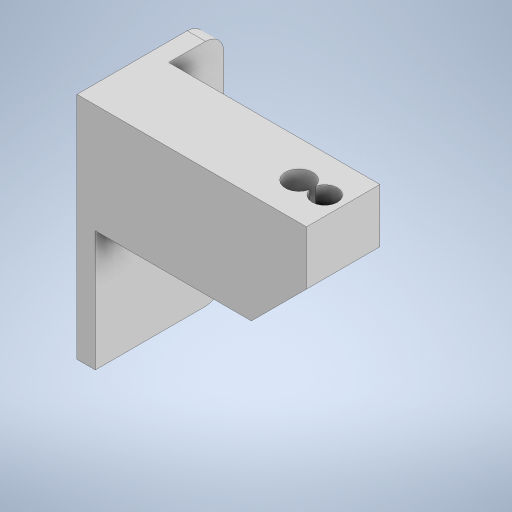
# Autodesk Inventor part: Futaba Antenna Mount
Saved by Autodesk Inventor 2024 (Build 280153000, 153)
## iProperties
Created: 2023-11-29
Part Number: Futaba Antenna Mount
Material: Generic
Document SubType Name: Modeling
Designer: close
Density: 1 g/cm^3
Appearance: Default
Author: close
Autodesk Inventor part; units mm, degrees
ref_plane "YZ Plane" through (0, 0, 0) normal (1, 0, 0) x (0, 1, 0)
ref_plane "XZ Plane" through (0, 0, 0) normal (0, 1, 0) x (-1, 0, 0)
ref_plane "XY Plane" through (0, 0, 0) normal (0, 0, 1) x (1, 0, 0)
sketch "Sketch1" plane through (0, 0, 0) normal (1, 0, 0) x (0, 1, 0)
  line L0 (0, 0) -> (25, 0)
  line L1 (25, 0) -> (25, -8)
  line L2 (25, -8) -> (0, -8)
  line L3 (0, -8) -> (0, 0)
  line L4 (25, -8) -> (12.5, -8)
  line L5 (12.5, -8) -> (12.5, -14)
  line L6 (12.5, -14) -> (25, -14)
  line L7 (25, -14) -> (25, -8)
  line L8 (0, -8) -> (12.5, -8)
  line L9 (12.5, -8) -> (12.5, -14)
  line L10 (12.5, -14) -> (0, -14)
  line L11 (0, -14) -> (0, -8)
  line L12 (25, 0) -> (13.125, 0)
  line L13 (13.125, 0) -> (13.125, -8)
  line L14 (13.125, -8) -> (25, -8)
  line L15 (25, -8) -> (25, 0)
  line L16 (19.5, -11) -> (5.5, -11) construction
  circle A0 centre (19.5, -11) radius 1.65
  circle A1 centre (5.5, -11) radius 1.65
  circle A2 centre (12.5, -11) radius 1.336701
  point P0 (12.5, -8)
  point P1 (25, -11)
  point P2 (12.5, -8)
  point P3 (12.5, -8)
  point P4 (13.125, 0)
  dimension "d0" = 0.625
  dimension "d1" = 14
  dimension "d2" = 25
  dimension "d3" = 12.5
  dimension "d4" = 12.5
  dimension "d6" = 3
  dimension "d7" = 0
  dimension "d8" = 8
  dimension "d11" = 3.3
  dimension "d12" = 3.3
  dimension "d28" = 5.5
  constraints: 34 end point, 8 parallel, 5 horizontal, 4 perpendicular, 3 centre point, 3 midpoint, 2 coincident, 1 collinear, 1 point on line
  measures "d0" distance from line of L13 point (12.5, -8)
  measures "d1" distance of L16.start L16.end
  measures "d2" distance between parallel lines of L3 L1
  measures "d3" distance between parallel lines of L7 L5
  measures "d4" distance between parallel lines of L11 L9
  measures "d6" distance from line of L16.start L6
  measures "d7" distance from line of point (25, -11) L16
  measures "d8" distance between parallel lines of L0 L2
  measures "d11" diameter of A0
  measures "d12" diameter of A1
  measures "d28" distance of point (25, -11) L16.start
sketch "Sketch1 outline for Extrusion1" plane through (0, 0, 0) normal (1, 0, 0) x (0, 1, 0)
  line L0 (0, 0) -> (0, -8)
  line L1 (25, 0) -> (0, 0)
  line L2 (0, -8) -> (0, -14)
  line L3 (25, -8) -> (25, 0)
  line L4 (0, -14) -> (12.5, -14)
  line L5 (25, -14) -> (25, -8)
  line L6 (12.5, -14) -> (25, -14)
  circle A0 centre (5.5, -11) radius 1.65
  circle A1 centre (12.5, -11) radius 1.336701
  circle A2 centre (19.5, -11) radius 1.65
extrude "Extrusion1" add sketch "Sketch1 outline for Extrusion1" along normal blind 2
fillet "Fillet1" radius 2 3 edges at (1, 25, -14) (1, 12.5, -14) (1, 0, -14)
sketch "Sketch1 outline for Extrusion2" plane through (0, 0, 0) normal (1, 0, 0) x (0, 1, 0)
  line L0 (13.125, 0) -> (13.125, -8)
  line L1 (25, 0) -> (13.125, 0)
  line L2 (25, -8) -> (25, 0)
  line L3 (13.125, -8) -> (25, -8)
extrude "Extrusion2" add sketch "Sketch1 outline for Extrusion2" along normal blind 25
chamfer "Chamfer1" distance 6 angle 45 1 edges at (25, 13.125, -4)
sketch "Sketch2" plane through (0, 25, 0) normal (0, 1, 0) x (1, 0, 0)
  line L0 (20.2, 4) -> (23, 4) construction
  line L1 (2, 8) -> (25, 8) projected
  line L2 (0, 0) -> (25, 0) projected
  circle A0 centre (20.2, 4) radius 1.5
  circle A1 centre (23, 4) radius 1.45
  circle A2 centre (23, 4) radius 1.375
  line L3 (25, 8) -> (25, 0) projected
  point P0 (2, 4.5)
  point P1 (21.664174, 3.674126)
  point P2 (21.664174, 4.325874)
  dimension "d19" = 8
  dimension "d20" = 4
  dimension "d21" = 3
  dimension "d22" = 2.9
  dimension "d23" = 2.75
  dimension "d24" = 2
  dimension "d25" = 2.8
  constraints: 5 coincident, 3 centre point, 2 end point, 1 horizontal, 1 other
  measures "d20" distance of the line from the sketch origin of L0
  measures "d21" diameter of A0
  measures "d22" diameter of A1
  measures "d23" diameter of A2
  measures "d24" distance from line of L3 L0.end
  measures "d25" distance of L0.start L0.end
sketch "Sketch2 outline for Extrusion3" plane through (0, 25, 0) normal (0, 1, 0) x (1, 0, 0)
  arc A0 (21.664174, 4.325874) -> (21.664174, 3.674126) centre (20.2, 4) ccw
  arc A1 (21.664174, 3.674126) -> (21.664174, 4.325874) centre (23, 4) ccw
extrude "Extrusion3" cut sketch "Sketch2 outline for Extrusion3" against normal blind 12.5
equation "\"d3\" = 0.5 * d2"
equation "\"d4\" = d3"
equation "\"d6\" = d5"
equation "\"d12\" = d11"
equation "\"d28\" = -0.5 * d1 + 0.5 * d2"
equation "\"d20\" = 0.5 * d19"
equation "\"d5\" = 3"
body "Solid1"
